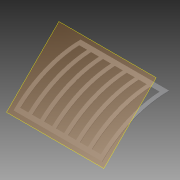
# Autodesk Inventor part: Back
Saved by Autodesk Inventor 2013 (Build 170138000, 138)
## iProperties
Created: 2013-01-27
Part Number: Back
Material: Polycarbonate, Clear
Document SubType Name: Modeling
Designer: Andrew Toennies
Density: 1.2 g/cm^3
Mass: 56.1141 g
Surface Area: 658.617 cm^2
Volume: 46.7618 cm^3
Author: Andrew Toennies
Autodesk Inventor part; units mm, degrees
ref_plane "YZ Plane" through (0, 0, 0) normal (1, 0, 0) x (0, 1, 0)
ref_plane "XZ Plane" through (0, 0, 0) normal (0, 1, 0) x (-1, 0, 0)
ref_plane "XY Plane" through (0, 0, 0) normal (0, 0, 1) x (1, 0, 0)
sketch "Sketch1" plane through (0, 0, 0) normal (1, 0, 0) x (0, 1, 0)
  arc A0 (301.625, 0) -> (213.2811, 213.2811) centre (0, 0) ccw
  arc A1 (303.2125, 0) -> (214.4036, 214.4036) centre (0, 0) ccw
  line L0 (0, 0) -> (471.039, 0)
  line L1 (0, 0) -> (335.2588, 335.2588)
  dimension "d0" = 603.25
  dimension "d1" = 1.5875
  dimension "d2" = 45
  constraints: 4 end point, 4 point on circle, 4 point on line, 2 centre point, 2 coincident, 1 horizontal
  measures "d0" diameter of A0
  measures "d1" radial gap between concentric circles of A1 A0
  measures "d2" angle of L0 L1
extrude "Extrusion1" add sketch "Sketch1" along normal blind 282.575 contours A0 L1 A1 L0
ref_plane "Work Plane2" through (0, 214.4036, 214.4036) normal (0, 0.7071, 0.7071) x (1, 0, 0)
ref_plane "Work Plane1" through (282.3966, 77.4773, 86.4575) normal (0, 0.7071, -0.7071) x (1, 0, 0)
sketch "Sketch2" plane through (0, 214.4036, 214.4036) normal (0, 0.7071, 0.7071) x (1, 0, 0)
  line L0 (0, 0) -> (0, 214.4014)
  line L1 (0, 214.4014) -> (282.575, 214.4014)
  line L2 (282.575, 214.4014) -> (282.575, 0)
  line L3 (282.575, 0) -> (0, 0)
  line L4 (269.875, 12.7) -> (269.875, 201.7014)
  line L5 (12.7, 201.7014) -> (12.7, 12.7)
  line L6 (38.1, 201.7014) -> (38.1, 12.7)
  line L7 (50.8, 201.7014) -> (50.8, 12.7)
  line L8 (76.2, 201.7014) -> (76.2, 12.7)
  line L9 (88.9, 201.7014) -> (88.9, 12.7)
  line L10 (114.3, 201.7014) -> (114.3, 12.7)
  line L11 (127, 201.7014) -> (127, 12.7)
  line L12 (152.4, 201.7014) -> (152.4, 12.7)
  line L13 (190.5, 201.7014) -> (190.5, 12.7)
  line L14 (165.1, 201.7014) -> (165.1, 12.7)
  line L15 (203.2, 201.7014) -> (203.2, 12.7)
  line L16 (228.6, 12.7) -> (228.6, 201.7014)
  line L17 (241.3, 12.7) -> (241.3, 201.7014)
  line L18 (38.1, 201.7014) -> (12.7, 201.7014)
  line L19 (76.2, 201.7014) -> (50.8, 201.7014)
  line L20 (114.3, 201.7014) -> (88.9, 201.7014)
  line L21 (152.4, 201.7014) -> (127, 201.7014)
  line L22 (190.5, 201.7014) -> (165.1, 201.7014)
  line L23 (269.875, 201.7014) -> (241.3, 201.7014)
  line L24 (228.6, 201.7014) -> (203.2, 201.7014)
  line L25 (241.3, 12.7) -> (269.875, 12.7)
  line L26 (203.2, 12.7) -> (228.6, 12.7)
  line L27 (165.1, 12.7) -> (190.5, 12.7)
  line L28 (127, 12.7) -> (152.4, 12.7)
  line L29 (88.9, 12.7) -> (114.3, 12.7)
  line L30 (12.7, 12.7) -> (38.1, 12.7)
  line L31 (50.8, 12.7) -> (76.2, 12.7)
  dimension "d6" = 214.4014
  dimension "d7" = 282.575
  dimension "d8" = 12.7
  dimension "d9" = 25.4
  dimension "d10" = 12.7
  dimension "d11" = 25.4
  dimension "d12" = 12.7
  dimension "d13" = 25.4
  dimension "d14" = 12.7
  dimension "d15" = 25.4
  dimension "d16" = 12.7
  dimension "d17" = 25.4
  dimension "d18" = 12.7
  dimension "d19" = 25.4
  dimension "d20" = 12.7
  constraints: 64 end point, 61 parallel, 29 perpendicular, 1 vertical
  measures "d6" distance of L0.start L0.end
  measures "d7" distance of L0.end L1.end
  measures "d8" distance between parallel lines of L2 L4
  measures "d9" distance between parallel lines of L5 L6
  measures "d10" distance between parallel lines of L6 L7
  measures "d11" distance between parallel lines of L8 L7
  measures "d12" distance between parallel lines of L8 L9
  measures "d13" distance between parallel lines of L10 L9
  measures "d14" distance between parallel lines of L11 L10
  measures "d15" distance between parallel lines of L12 L11
  measures "d16" distance between parallel lines of L14 L12
  measures "d17" distance between parallel lines of L13 L14
  measures "d18" distance between parallel lines of L15 L13
  measures "d19" distance between parallel lines of L15 L16
  measures "d20" distance between parallel lines of L17 L16
extrude "Extrusion2" cut sketch "Sketch2" against normal blind 4826000 contours L25 L17 L23 L4 | L18 L6 L30 L5 | L19 L8 L31 L7 | L20 L10 L29 L9 | L21 L12 L28 L11 | L13 L27 L14 L22 | L24 L16 L26 L15
body "Solid1"
